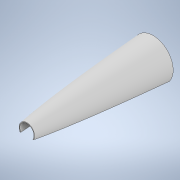
# Autodesk Inventor part: nose-toppart1
Saved by Autodesk Inventor 2020.3 (Build 243373000, 373)
## iProperties
Created: 2021-03-10
Part Number: nose-toppart1
Material: Generic
Document SubType Name: Modeling
Designer: 0x6f736f646f
Density: 1 g/cm^3
Appearance: Default
Author: 0x6f736f646f
Autodesk Inventor part; units mm, degrees
ref_plane "YZ Plane" through (0, 0, 0) normal (1, 0, 0) x (0, 1, 0)
ref_plane "XZ Plane" through (0, 0, 0) normal (0, 1, 0) x (-1, 0, 0)
ref_plane "XY Plane" through (0, 0, 0) normal (0, 0, 1) x (1, 0, 0)
sketch "Sketch3" plane through (0, 0, 0) normal (1, 0, 0) x (0, 1, 0)
  line L0 (0, 0) -> (25, 0)
  line L1 (25, 0) -> (25, -5)
  line L2 (25, -5) -> (26.8, -5)
  line L3 (26.8, -5) -> (26.8, 0)
  line L4 (0, 0) -> (-25, 0)
  line L5 (0, 0) -> (0, 200)
  line L6 (-25, 0) -> (-26.8, 0)
  spline S0 degree 2 poles (26.8, 0) (13.4, 200) (0, 200) knots 0 0 0 0.5 0.5 0.5
  line L7 (0, 0) -> (0, 198.2)
  spline S1 degree 2 poles (25, 0) (12.5, 198.2) (0, 198.2) knots 0 0 0 0.5 0.5 0.5
  line L8 (0, 2) -> (26.6657, 2)
  line L9 (0, 170) -> (0, 0)
  line L10 (0, 0) -> (0, 170)
  line L11 (0, 170) -> (10.3796, 170)
  line L12 (0, 172) -> (10.0276, 172)
  line L13 (1.8152, 198.2) -> (-1.8152, 198.2) construction
  arc A0 (1.0681, 197.7831) -> (-1.0681, 197.7831) centre (0, 196.6233) ccw construction
  line L14 (1.9566, 200) -> (-1.9566, 200) construction
  arc A1 (1.1799, 199.5579) -> (-1.1799, 199.5579) centre (0, 198.2044) ccw construction
  line L15 (0, 0) -> (-6, 0)
  line L16 (0, 170) -> (0, 0)
  line L17 (0, 2) -> (-5, 2)
  line L18 (-5, 2) -> (-5, 170)
  line L19 (-5, 170) -> (0, 170)
  line L20 (0, 170) -> (0, 2)
  line L21 (-5, 2) -> (-15, 2)
  line L22 (-15, 2) -> (-5, 170)
  spline S2 degree 2 poles (26.8, 0) (0, 400) (-26.8, 0) knots 0 0 0 1 1 1
  spline S3 degree 2 poles (-25, 0) (0, 396.4088) (25, 0) knots 0 0 0 1 1 1
  point P0 (9.0895, 172)
  point P1 (0, 172)
  point P2 (0, 170)
  point P3 (9.43, 170)
  point P4 (24.8735, 2)
  point P5 (0, 170)
  point P6 (9.43, 170)
  point P7 (24.8735, 2)
  point P8 (0, 170)
  dimension "d24" = 25
  dimension "d25" = 5
  dimension "d26" = 1.8
  dimension "d27" = 25
  dimension "d28" = 200
  dimension "d29" = 1.8
  dimension "d30" = 198.2
  dimension "d31" = 2
  dimension "d32" = 5
  dimension "d33" = 10
  constraints: 46 end point, 10 horizontal, 4 midpoint, 3 parallel, 3 perpendicular, 3 point on line, 2 centre point, 2 collinear, 2 point on circle, 2 vertical, 15 other
  measures "d24" distance of L0.start L0.end
  measures "d25" distance of L0.end L1.end
  measures "d26" distance of L1.end L2.end
  measures "d27" distance of L0.start L4.end
  measures "d28" distance of L5.end L0.start
  measures "d29" distance of L4.end L6.end
  measures "d30" distance of L7.end L0.start
  measures "d31" distance between parallel lines of L11 L12
  measures "d32" distance of L18.end L19.end
  measures "d33" distance of L17.end L21.end
revolve "Revolution3" add sketch "Sketch3" angle 360 mid plane about axis through (0, 0, 170) along (0, 0, -1) contours S1 L11 S0 L8
extrude "Extrusion3" cut sketch "Sketch3" against normal mid plane 60 contours L4 S3 L5 L19 L22 L21 L17 | L6 S2 L5 S3
body "Solid2"
